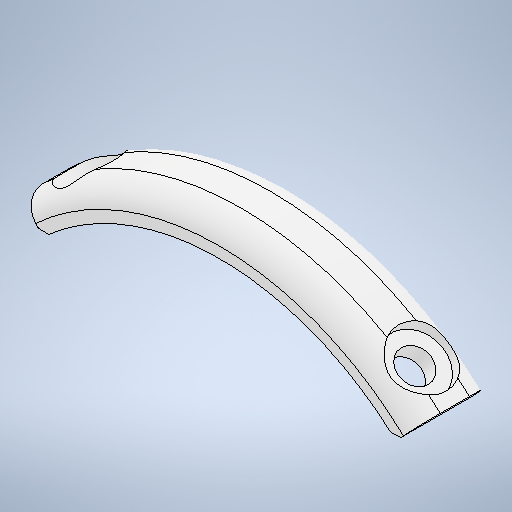
# Autodesk Inventor part: joint4_base_support_fixture
Saved by Autodesk Inventor 2025.3 (Build 293356030, 356C)
## iProperties
Created: 2025-11-09
Part Number: joint4_base_support_fixture
Material: PLA filament
Document SubType Name: Modeling
Designer: MSI
Mass: 2.45003 g
Surface Area: 16.4298 cm^2
Volume: 2.04169 cm^3
Density: 1.2 g/cm^3
Appearance: 일반
Author: MSI
Autodesk Inventor part; units mm, degrees
ref_plane "YZ Plane" through (0, 0, 0) normal (1, 0, 0) x (0, 1, 0)
ref_plane "XZ Plane" through (0, 0, 0) normal (0, 1, 0) x (-1, 0, 0)
sketch "스케치1" plane through (0, 0, 0) normal (0, 0, 1) x (1, 0, 0)
  arc A0 (27.279934, 29.254148) -> (-27.279934, 29.254148) centre (0, 0) ccw
  line L0 (-27.279934, 29.254148) -> (0, 0)
  line L1 (0, 0) -> (27.279934, 29.254148)
  line L2 (0, 0) -> (0, 40)
  circle A1 centre (0, 0) radius 35.5
  point P0 (24.210942, 25.963056)
  point P1 (-24.210942, 25.963056)
  dimension "d1" = 40
  dimension "d2" = 43
  dimension "d3" = 43
  dimension "d4" = 4.5
  constraints: 6 end point, 3 point on circle, 2 centre point, 2 coincident, 1 vertical
  measures "d1" radius of A0
  measures "d2" angle of L2 L0
  measures "d3" angle of L2 L1
  measures "d4" radial gap between concentric circles of A0 A1
extrude "돌출1" add sketch "스케치1" along normal mid plane 10 contours L1 A1 L2 A0 | L2 A1 L0 A0
sketch "스케치2" plane through (0, 0, 0) normal (0, 0, 1) x (1, 0, 0)
  line L0 (0, 0) -> (-22.943057, 32.766082)
  arc A0 (27.279934, 29.254148) -> (-27.279934, 29.254148) centre (0, 0) ccw
  line L1 (0, 0) -> (0, 40.096448) construction
  dimension "d7" = 35
  constraints: 4 end point, 1 point on circle, 1 vertical
  measures "d7" angle of L0 L1
ref_plane "작업 평면1" through (-22.943057, 32.766082, 0) normal (-0.5735764, 0.819152, 0) x (-0.819152, -0.5735764, 0)
sketch "스케치3" plane through (-22.943057, 32.766082, 0) normal (-0.5735764, 0.819152, 0) x (-0.819152, -0.5735764, 0)
  point P0 (0, 0)
  point P1 (0, 0)
  constraints: 1 coincident
hole "구멍1" at (-22.943057, 32.766082, 0) direction (0.5735764, -0.819152, 0) diameter 4.5 end through all counterbore diameter 8 counterbore depth 2 clearance for "Socket Head Cap Screw ISO 4762" size "M4" standard "ISO"
mirror "미러1" about plane through (0, 0, 0) normal (1, 0, 0) of "구멍1"
fillet "모깎기1" radius 3 2 edges at (0, 40, 5) (0, 40, -5)
chamfer "모따기1" distance 1 angle 45 2 edges at (24.2109, 25.9631, 0) (-24.2109, 25.9631, 0)
equation "\"d3\" = d2"
